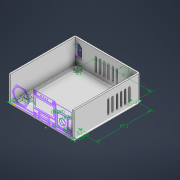
# Autodesk Inventor part: Part1
Saved by Autodesk Inventor 2021 (Build 250183000, 183)
## iProperties
Created: 2022-12-02
Part Number: Part1
Material: Generic
Document SubType Name: Modeling
Designer: Martin Adytia
Density: 1 g/cm^3
Appearance: Default
Author: Martin Adytia
Autodesk Inventor part; units mm, degrees
ref_plane "YZ Plane" through (0, 0, 0) normal (1, 0, 0) x (0, 1, 0)
ref_plane "XZ Plane" through (0, 0, 0) normal (0, 1, 0) x (-1, 0, 0)
ref_plane "XY Plane" through (0, 0, 0) normal (0, 0, 1) x (1, 0, 0)
sketch "Sketch1" plane through (0, 0, 0) normal (0, 1, 0) x (-1, 0, 0)
  line L0 (0, 0) -> (-70, 0)
  line L1 (-70, 0) -> (-70, -67.3)
  line L2 (-70, -67.3) -> (0, -67.3)
  line L3 (0, -67.3) -> (0, 0)
  line L4 (-70, -67.3) -> (-70, -64.3)
  circle A0 centre (-67, -64.3) radius 1.55
  line L5 (0, -67.3) -> (0, -64.3)
  line L6 (0, -64.3) -> (-2, -64.3)
  circle A1 centre (-2, -64.3) radius 1.55
  line L7 (0, 0) -> (4, 0)
  line L8 (-70, 0) -> (-70, 9)
  line L9 (-70, -67.3) -> (-71, -67.3)
  line L10 (-71, -67.3) -> (-71, 9)
  line L11 (-71, 9) -> (-70, 9)
  line L12 (-70, 9) -> (-70, -67.3)
  line L13 (-71, -67.3) -> (0, -67.3)
  line L14 (0, -67.3) -> (0, -68.3)
  line L15 (0, -68.3) -> (-71, -68.3)
  line L16 (-71, -68.3) -> (-71, -67.3)
  line L17 (4, 0) -> (5, 0)
  line L18 (5, 0) -> (5, -68.3)
  line L19 (5, -68.3) -> (4, -68.3)
  line L20 (4, -68.3) -> (4, 0)
  line L21 (0, -67.3) -> (4, -67.3)
  line L22 (4, -68.3) -> (0, -68.3)
  line L23 (-71, 9) -> (5, 9)
  line L24 (5, 9) -> (5, 8)
  line L25 (5, 8) -> (-71, 8)
  line L26 (-71, 8) -> (-71, 9)
  line L27 (5, 0) -> (4, 0)
  line L28 (4, 0) -> (4, 8)
  line L29 (4, 8) -> (5, 8)
  line L30 (5, 8) -> (5, 0)
  line L31 (5, -68.3) -> (-71, -68.3)
  line L32 (-71, -68.3) -> (-71, -70.3)
  line L33 (-71, -70.3) -> (5, -70.3)
  line L34 (5, -70.3) -> (5, -68.3)
  line L35 (-71, -70.3) -> (-73, -70.3)
  line L36 (-73, -70.3) -> (-73, 9)
  line L37 (-73, 9) -> (-71, 9)
  line L38 (-71, 9) -> (-71, -70.3)
  line L39 (-73, 9) -> (5, 9)
  line L40 (5, 9) -> (5, 11)
  line L41 (5, 11) -> (-73, 11)
  line L42 (-73, 11) -> (-73, 9)
  line L43 (5, 11) -> (7, 11)
  line L44 (7, 11) -> (7, -70.3)
  line L45 (7, -70.3) -> (5, -70.3)
  line L46 (5, -70.3) -> (5, 11)
  circle A2 centre (-2, -64.3) radius 3
  circle A3 centre (-67, -64.3) radius 3
  circle A4 centre (-66.9693, -3.0346) radius 1.55
  circle A5 centre (-66.9693, -3.0346) radius 3
  circle A6 centre (-2.0948, -2.9942) radius 1.55
  circle A7 centre (-2.0948, -2.9942) radius 3
  point P0 (-69, -63.3)
  dimension "d0" = 70
  dimension "d1" = 67.3
  dimension "d2" = 3
  dimension "d3" = 3.1
  dimension "d4" = 3
  dimension "d5" = 2
  dimension "d6" = 3.1
  dimension "d7" = 4
  dimension "d8" = 9
  dimension "d9" = 1
  dimension "d10" = 1
  dimension "d11" = 1
  dimension "d12" = 1
  dimension "d13" = 2
  dimension "d14" = 2
  dimension "d15" = 2
  dimension "d16" = 2
  dimension "d62" = 3.1
  dimension "d63" = 6
  dimension "d64" = 3.1
  dimension "d65" = 6
  constraints: 94 end point, 21 parallel, 12 perpendicular, 11 horizontal, 7 centre point, 7 point on line, 5 coincident, 1 horizontal alignment, 1 vertical, 2 other
  measures "d0" distance of L2.end L1.end
  measures "d1" distance of L1.end L0.end
  measures "d2" distance of L1.end L4.end
  measures "d3" diameter of A0
  measures "d4" distance of L2.end L5.end
  measures "d5" distance of L5.end L6.end
  measures "d6" diameter of A1
  measures "d7" distance of L0.start L7.end
  measures "d8" distance of L0.end L8.end
  measures "d9" distance of L10.end L11.end
  measures "d10" distance of L13.end L14.end
  measures "d11" distance of L18.end L19.end
  measures "d12" distance of L23.end L24.end
  measures "d13" distance of L32.end L31.end
  measures "d14" distance of L36.end L37.end
  measures "d15" distance of L40.end L39.end
  measures "d16" distance of L44.end L45.end
  measures "d62" diameter of A4
  measures "d63" diameter of A5
  measures "d64" diameter of A6
  measures "d65" diameter of A7
extrude "Extrusion2" add sketch "Sketch1" against normal blind 2 contours L3 A7 L0 | L7 L20 L21 L3 A2 A7 | L0 A7 L8 L25 L28 L7 | A7 L3 L0 | L0 A7 | A7 L3 | L28 L25 L30 L17 | L17 L18 L19 L20 | A7 L3 A2 L2 A3 L1 L0 | L30 L24 L40 L43 L44 L45 L34 L18 | L20 L22 L14 L21 | L25 L8 L23 L24 | L1 L9 L10 L25 L8 | A2 L3 | L3 A2 | L34 L33 L32 L15 L22 L19 | L14 L15 L16 L9 L2 | L2 A2 L3 | L25 L10 L11 L8 | A3 L2 L1 | A3 | L23 L11 L37 L42 L41 L40 | L10 L16 L32 L35 L36 L37 | A0 | A1 | A4 | A5 | A6
extrude "Extrusion3" add sketch "Sketch1" along normal blind 3 contours A2 L3 | L3 A2 | A3
extrude "Extrusion4" cut sketch "Sketch1" against normal blind 1 contours A0 | A1
fillet "Fillet1" radius 1 1 edges at (70, 0, -64.3)
fillet "Fillet2" radius 1 1 edges at (5, 0, -64.3)
extrude "Extrusion5" add sketch "Sketch1" along normal blind 30 contours L30 L24 L40 L43 L44 L45 L34 L18 | L34 L33 L32 L15 L22 L19 | L23 L11 L37 L42 L41 L40 | L10 L16 L32 L35 L36 L37
sketch "Sketch2" plane through (-7, -2, 11) normal (0, 0, 1) x (1, 0, 0)
  line L0 (71.2558, 20.3181) -> (59.4702, 20.3181)
  line L1 (59.4702, 20.3181) -> (59.4702, 18.5401)
  line L2 (59.4702, 15.3651) -> (59.4702, 10.5391)
  line L3 (59.4702, 7.3641) -> (59.4702, 6.6021)
  line L4 (59.4702, 6.6021) -> (71.2558, 6.6021)
  line L5 (71.2558, 6.6021) -> (71.2558, 7.3641)
  line L6 (71.2558, 10.5391) -> (71.2558, 15.3651)
  line L7 (71.2558, 18.5401) -> (71.2558, 20.3181)
  line L8 (77.0216, 28.7521) -> (57.6922, 28.7521)
  line L9 (57.6922, 28.7521) -> (57.6922, 2.3361)
  line L10 (57.6922, 2.3361) -> (77.0216, 2.3361)
  line L11 (77.0216, 2.3361) -> (77.0216, 28.7521)
  circle A0 centre (74.5578, 22.0211) radius 1.5
  circle A1 centre (74.5578, 8.1019) radius 1.5
  circle A2 centre (65.363, 12.9521) radius 3.4544
  line L12 (54.1324, 12.5617) -> (54.1324, 23.7817)
  line L13 (54.1324, 23.7817) -> (32.5724, 23.7817)
  line L14 (32.5724, 23.7817) -> (32.5724, 12.5617)
  line L15 (32.5724, 12.5617) -> (54.1324, 12.5617)
  line L16 (56.1024, 10.9717) -> (56.1024, 25.3717)
  line L17 (56.1024, 25.3717) -> (30.6024, 25.3717)
  line L18 (30.6024, 25.3717) -> (30.6024, 10.9717)
  line L19 (30.6024, 10.9717) -> (56.1024, 10.9717)
  line L20 (54.1324, 23.7817) -> (54.1324, 12.5617)
  line L21 (54.1324, 12.5617) -> (32.5724, 12.5617)
  line L22 (32.5724, 12.5617) -> (32.5724, 23.7817)
  line L23 (32.5724, 23.7817) -> (54.1324, 23.7817)
  line L24 (35.8555, 8.9917) -> (49.8555, 8.9917)
  line L25 (49.8555, 8.9917) -> (49.8555, 7.9917)
  line L26 (49.8555, 7.9917) -> (47.8555, 7.9917)
  line L27 (47.8555, 7.9917) -> (47.8554, 6.6117)
  line L28 (47.8554, 6.6117) -> (56.6024, 6.6117)
  line L29 (56.6024, 25.8717) -> (56.6024, 6.6117)
  line L30 (30.1024, 25.8717) -> (56.6024, 25.8717)
  line L31 (30.1024, 6.6117) -> (30.1024, 25.8717)
  line L32 (30.1024, 6.6117) -> (37.8601, 6.6117)
  line L33 (37.8601, 6.6117) -> (37.8601, 7.9917)
  line L34 (37.8601, 7.9917) -> (35.8555, 7.9917)
  line L35 (35.8555, 7.9917) -> (35.8555, 8.9917)
  line L36 (30.6024, 25.3717) -> (56.1024, 25.3717)
  line L37 (56.1024, 25.3717) -> (56.1024, 10.9717)
  line L38 (56.1024, 10.9717) -> (30.6024, 10.9717)
  line L39 (30.6024, 10.9717) -> (30.6024, 25.3717)
  arc A3 (31.8024, 2.3117) -> (30.0024, 4.1117) centre (31.8024, 4.1117) ccw
  line L40 (31.8024, 2.3117) -> (35.8555, 2.3117)
  line L41 (35.8555, 2.3117) -> (35.8555, 4.3117)
  line L42 (49.8555, 4.3117) -> (35.8555, 4.3117)
  line L43 (49.8555, 4.3117) -> (49.8555, 2.3117)
  line L44 (49.8555, 2.3117) -> (54.9024, 2.3117)
  arc A4 (56.7024, 4.1117) -> (54.9024, 2.3117) centre (54.9024, 4.1117) ccw
  line L45 (56.7024, 30.1717) -> (56.7024, 4.1117)
  line L46 (30.0024, 30.1717) -> (56.7024, 30.1717)
  line L47 (30.0024, 30.1717) -> (30.0024, 4.1117)
  circle A5 centre (42.0824, 27.8217) radius 0.5
  circle A6 centre (44.6224, 27.8217) radius 0.5
  circle A7 centre (47.1624, 27.8217) radius 0.5
  circle A8 centre (39.5424, 27.8217) radius 0.5
  circle A9 centre (54.9024, 27.6717) radius 1
  circle A10 centre (31.8024, 27.6717) radius 1
  line L48 (56.6024, 10.3717) -> (56.6024, 25.8717)
  line L49 (30.1024, 10.3717) -> (56.6024, 10.3717)
  line L50 (30.1024, 25.8717) -> (30.1024, 10.3717)
  line L51 (56.6024, 25.8717) -> (30.1024, 25.8717)
  circle A11 centre (31.8024, 4.1117) radius 1.8
  line L52 (30.0024, 2.3117) -> (31.8024, 2.3117)
  line L53 (30.0024, 4.1117) -> (30.0024, 2.3117)
  line L54 (54.9024, 2.3117) -> (56.7024, 2.3117)
  line L55 (56.7024, 4.1117) -> (56.7024, 2.3117)
  circle A12 centre (54.9024, 4.1117) radius 1.8
  circle A13 centre (54.9024, 27.6717) radius 1.8
  circle A14 centre (31.8024, 27.6717) radius 1.8
  line L56 (37.8601, 6.6117) -> (37.8601, 2.3117)
  line L57 (47.8554, 6.6117) -> (37.8601, 6.6117)
  line L58 (37.8601, 6.6117) -> (37.8601, 2.3117)
  line L59 (47.8554, 2.3117) -> (37.8601, 2.3117)
  line L60 (47.8554, 2.3117) -> (47.8554, 6.6117)
  line L61 (36.8554, 6.6117) -> (36.8554, 2.3318)
  line L62 (36.8554, 2.3318) -> (48.8554, 2.3318)
  line L63 (48.8554, 2.3318) -> (48.8554, 6.6117)
  line L64 (48.8554, 6.6117) -> (36.8554, 6.6117)
  line L65 (48.8554, 2.3318) -> (48.8554, 6.6117)
  circle A15 centre (14.6189, 15.1235) radius 9.5
  circle A16 centre (14.6189, 15.1235) radius 8.4463
  line L66 (7.7436, 8.0317) -> (5.0396, 12.7153)
  line L67 (17.3229, 5.6235) -> (11.9148, 5.6235)
  line L68 (9.1386, 5.6235) -> (11.9148, 5.6235)
  line L69 (7.7436, 8.0317) -> (9.1317, 5.6275)
  line L70 (20.106, 5.6275) -> (21.4941, 8.0317)
  line L71 (17.3229, 5.6235) -> (20.0991, 5.6235)
  line L72 (24.1981, 12.7153) -> (21.4941, 8.0317)
  line L73 (24.1981, 12.7153) -> (25.5862, 15.1195)
  line L74 (25.5862, 15.1275) -> (24.1981, 17.5317)
  line L75 (21.4941, 22.2153) -> (24.1981, 17.5317)
  line L76 (21.4941, 22.2153) -> (20.106, 24.6195)
  line L77 (20.0991, 24.6235) -> (17.3229, 24.6235)
  line L78 (11.9148, 24.6235) -> (17.3229, 24.6235)
  line L79 (11.9148, 24.6235) -> (9.1386, 24.6235)
  line L80 (9.1317, 24.6195) -> (7.7436, 22.2153)
  line L81 (5.0396, 17.5317) -> (7.7436, 22.2153)
  line L82 (5.0396, 17.5317) -> (3.6515, 15.1275)
  line L83 (3.6515, 15.1195) -> (5.0396, 12.7153)
  line L84 (59.4702, 20.3181) -> (59.4702, 20.8181)
  line L85 (59.4702, 20.3181) -> (59.9702, 20.3181) construction
  line L86 (71.2558, 20.3181) -> (71.7558, 20.3181)
  line L87 (71.2558, 20.3181) -> (71.7558, 20.3181) construction
  line L88 (71.2558, 6.6021) -> (71.2558, 6.1021)
  line L89 (59.4702, 6.6021) -> (58.9702, 6.6021)
  line L90 (59.4702, 20.8181) -> (71.7558, 20.8181)
  line L91 (71.7558, 20.8181) -> (71.7558, 6.1021)
  line L92 (71.7558, 6.1021) -> (58.9702, 6.1021)
  line L93 (58.9702, 6.1021) -> (58.9702, 20.8181)
  line L94 (58.9702, 20.8181) -> (59.4702, 20.8181)
  circle A17 centre (65.363, 12.9521) radius 3.8
  line L95 (71.2558, 18.5401) -> (71.2558, 15.3651)
  line L96 (71.2558, 10.5391) -> (71.2558, 7.3641)
  line L97 (59.4702, 10.5391) -> (59.4702, 7.3641)
  line L98 (59.4702, 18.5401) -> (59.4702, 15.3651)
  line L99 (57.6922, 22.6169) -> (73.0578, 22.6169)
  line L100 (73.0578, 22.6169) -> (73.0578, 4.7047)
  line L101 (73.0578, 4.7047) -> (57.6922, 4.7047)
  line L102 (57.6922, 4.7047) -> (57.6922, 22.6169)
  circle A18 centre (31.8024, 4.1117) radius 1
  circle A19 centre (54.9024, 4.1117) radius 1
  point P0 (7, 2)
  point P1 (45.1104, -3.166)
  point P2 (36.8554, 4.3117)
  point P3 (48.8554, 4.3117)
  point P4 (37.8601, 2.3318)
  point P5 (47.8554, 2.3318)
  dimension "d31" = 0.5
  dimension "d32" = 90
  dimension "d33" = 0.5
  dimension "d34" = 0
  dimension "d35" = 0.5
  dimension "d36" = 0.5
  dimension "d37" = 7.6
  constraints: 206 end point, 20 centre point, 6 horizontal, 5 perpendicular, 4 coincident, 4 point on circle, 3 collinear, 3 parallel, 2 equal length, 2 point on line, 2 vertical
  measures "d31" distance of L0.end L84.end
  measures "d32" angle of L85 L84
  measures "d33" distance of L0.start L86.end
  measures "d34" distance between parallel lines of L86 L87
  measures "d35" distance of L4.end L88.end
  measures "d36" distance of L3.end L89.end
  measures "d37" diameter of A17
extrude "Extrusion6" cut sketch "Sketch2" against normal blind 10 contours A16
extrude "Extrusion7" cut sketch "Sketch2" against normal blind 10 contours A2 | A17
extrude "Extrusion8" add sketch "Sketch2" against normal blind 8 contours L86 L91 L92 L88 L5 L96 L6 L95 L7 | L0 L84 L90 L91 L86 | L1 L98 L2 L97 L3 L89 L93 L94 L84 | L92 L93 L89 L4 L88 | L99 L100 L101 L9
extrude "Extrusion9" cut sketch "Sketch2" against normal blind 8 contours L15 L14 L13 L12 | L19 L18 L17 L16
extrude "Extrusion13" add sketch "Sketch2" against normal blind 5 contours L15 L14 L13 L12 | L19 L18 L17 L16 | L35 L34 L33 L32 L31 L49 L29 L28 L27 L26 L25 L24 | L24 L25 L26 L27 L57 L33 L34 L35 | L56 L42 L61 L32 | L57 L60 L42 L56 | L28 L63 L42 L60 | L61 L42 L41 L40 A3 L47 A14 L30 L31 L32 | L56 L62 L61 L42 | L42 L60 L62 L56 | L28 L29 L30 A13 L45 A4 L44 L43 L42 L63 | L42 L63 L62 L60 | L62 L60 L59 L56 | L31 L30 L29 L49 | A14 L47 L46 L45 A13 L30 | A14 | A11 A3 | L52 L53 A11 | A13 | A12 L55 L54 | A4 A12 | A5 | A6 | A7 | A8 | A9 | A10 | A18 | A19
extrude "Extrusion14" cut sketch "Sketch2" against normal blind 5 contours L15 L14 L13 L12 | L19 L18 L17 L16
extrude "Extrusion15" cut sketch "Sketch2" against normal blind 5 contours A9
extrude "Extrusion16" cut sketch "Sketch2" against normal blind 5 contours A10 | A18 | A19
extrude "Extrusion17" add sketch "Sketch2" against normal blind 2 contours A9 | A10 | A18 | A19
sketch "Sketch3" plane through (0, 30, 0) normal (0, 1, 0) x (1, 0, 0)
  line L0 (71, -9) -> (71, 64.3) projected
  line L1 (-5, -11) -> (71, -11)
  line L2 (71, -11) -> (71, 0)
  line L3 (71, 0) -> (-5, 0)
  line L4 (-5, 0) -> (-5, -11)
  point P0 (0, 0)
  constraints: 8 end point, 2 parallel, 1 horizontal, 1 perpendicular, 1 point on line
extrude "Extrusion18" cut sketch "Sketch3" against normal blind 30
extrude "Extrusion19" add sketch "Sketch1" along normal blind 3 contours A7 L3 L0 | L0 A7 | A7 L3 | A4 | A5 | A6 picked at (-0.1816, -2.9942)
extrude "Extrusion20" cut sketch "Sketch1" along normal blind 3 contours A6
extrude "Extrusion21" cut sketch "Sketch1" against normal blind 1 contours A6
extrude "Extrusion22" cut sketch "Sketch1" along normal blind 3 contours A4
extrude "Extrusion23" cut sketch "Sketch1" against normal blind 1 contours A4
fillet "Fillet3" radius 2 2 edges at (5.0948, 0, -2.9942) (69.9693, 0, -3.0346)
sketch "Sketch4" plane through (73, -2, -70.3) normal (0, 0, -1) x (-1, 0, 0)
  line L0 (77.9837, 11.3959) -> (77.9837, 23.7773)
  arc A0 (77.9837, 23.7773) -> (77.9105, 23.9541) centre (77.7337, 23.7773) ccw
  line L1 (77.9105, 23.9541) -> (75.0569, 26.8076)
  arc A1 (75.0569, 26.8076) -> (74.8801, 26.8809) centre (74.8801, 26.6309) ccw
  line L2 (74.8801, 26.8809) -> (72.9592, 26.8809)
  line L3 (72.7825, 26.8076) -> (69.8557, 23.8809)
  arc A2 (72.9592, 26.8809) -> (72.7825, 26.8076) centre (72.9592, 26.6309) ccw
  line L4 (70.1057, 11.1459) -> (77.7337, 11.1459)
  arc A3 (77.7337, 11.1459) -> (77.9837, 11.3959) centre (77.7337, 11.3959) ccw
  arc A4 (69.8557, 11.3959) -> (70.1057, 11.1459) centre (70.1057, 11.3959) ccw
  line L5 (69.8557, 23.8809) -> (69.8557, 11.3959)
  line L6 (80, 0) -> (80, 32) projected
  line L7 (80, 21.6857) -> (78, 21.6857)
  line L8 (78, 2) -> (78, 32) projected
  line L9 (37, 24) -> (37, 24)
  line L10 (38, 23) -> (38, 8)
  line L11 (37, 7) -> (37, 7)
  line L12 (36, 8) -> (36, 23)
  line L13 (42, 24) -> (42, 24)
  line L14 (43, 23) -> (43, 8)
  line L15 (42, 7) -> (42, 7)
  line L16 (41, 8) -> (41, 23)
  line L17 (47.2198, 23.9651) -> (47.2198, 23.9651)
  line L18 (48.2198, 22.9651) -> (48.2198, 7.9651)
  line L19 (47.2198, 6.9651) -> (47.2198, 6.9651)
  line L20 (46.2198, 7.9651) -> (46.2198, 22.9651)
  line L21 (52.2198, 23.9651) -> (52.2198, 23.9651)
  line L22 (53.2198, 22.9651) -> (53.2198, 7.9651)
  line L23 (52.2198, 6.9651) -> (52.2198, 6.9651)
  line L24 (51.2198, 7.9651) -> (51.2198, 22.9651)
  line L25 (32.3855, 23.0054) -> (32.3855, 8.0054)
  line L26 (31.3855, 24.0054) -> (31.3855, 24.0054)
  line L27 (31.3855, 7.0054) -> (31.3855, 7.0054)
  line L28 (30.3855, 8.0054) -> (30.3855, 23.0054)
  line L29 (27.3855, 23.0054) -> (27.3855, 8.0054)
  line L30 (26.3855, 24.0054) -> (26.3855, 24.0054)
  line L31 (26.3855, 7.0054) -> (26.3855, 7.0054)
  line L32 (25.3855, 8.0054) -> (25.3855, 23.0054)
  arc A5 (26.3855, 24.0054) -> (25.3855, 23.0054) centre (26.3855, 23.0054) ccw
  arc A6 (27.3855, 23.0054) -> (26.3855, 24.0054) centre (26.3855, 23.0054) ccw
  arc A7 (25.3855, 8.0054) -> (26.3855, 7.0054) centre (26.3855, 8.0054) ccw
  arc A8 (26.3855, 7.0054) -> (27.3855, 8.0054) centre (26.3855, 8.0054) ccw
  arc A9 (30.3855, 8.0054) -> (31.3855, 7.0054) centre (31.3855, 8.0054) ccw
  arc A10 (31.3855, 7.0054) -> (32.3855, 8.0054) centre (31.3855, 8.0054) ccw
  arc A11 (32.3855, 23.0054) -> (31.3855, 24.0054) centre (31.3855, 23.0054) ccw
  arc A12 (31.3855, 24.0054) -> (30.3855, 23.0054) centre (31.3855, 23.0054) ccw
  arc A13 (37, 24) -> (36, 23) centre (37, 23) ccw
  arc A14 (38, 23) -> (37, 24) centre (37, 23) ccw
  arc A15 (36, 8) -> (37, 7) centre (37, 8) ccw
  arc A16 (37, 7) -> (38, 8) centre (37, 8) ccw
  arc A17 (41, 8) -> (42, 7) centre (42, 8) ccw
  arc A18 (42, 7) -> (43, 8) centre (42, 8) ccw
  arc A19 (43, 23) -> (42, 24) centre (42, 23) ccw
  arc A20 (42, 24) -> (41, 23) centre (42, 23) ccw
  arc A21 (47.2198, 23.9651) -> (46.2198, 22.9651) centre (47.2198, 22.9651) ccw
  arc A22 (48.2198, 22.9651) -> (47.2198, 23.9651) centre (47.2198, 22.9651) ccw
  arc A23 (46.2198, 7.9651) -> (47.2198, 6.9651) centre (47.2198, 7.9651) ccw
  arc A24 (47.2198, 6.9651) -> (48.2198, 7.9651) centre (47.2198, 7.9651) ccw
  arc A25 (51.2198, 7.9651) -> (52.2198, 6.9651) centre (52.2198, 7.9651) ccw
  arc A26 (52.2198, 6.9651) -> (53.2198, 7.9651) centre (52.2198, 7.9651) ccw
  arc A27 (53.2198, 22.9651) -> (52.2198, 23.9651) centre (52.2198, 22.9651) ccw
  arc A28 (52.2198, 23.9651) -> (51.2198, 22.9651) centre (52.2198, 22.9651) ccw
  point P0 (73, 2)
  point P1 (73.9221, 19.0174)
  point P2 (41, 24)
  point P3 (43, 7)
  point P4 (51.2198, 23.9651)
  point P5 (53.2198, 6.9651)
  point P6 (32.3855, 7.0054)
  point P7 (30.3855, 24.0054)
  point P8 (52.2198, 6.9651)
  point P9 (42, 7)
  point P10 (37, 7)
  point P11 (31.3855, 24.0054)
  point P12 (31.3855, 7.0054)
  point P13 (26.3855, 7.0054)
  dimension "d77" = 2
  dimension "d80" = 1
  constraints: 62 end point, 58 point on circle, 48 tangent, 29 centre point, 23 equal radius, 20 point on line, 12 parallel, 6 horizontal, 6 perpendicular
  measures "d77" distance of L7.start L7.end
  measures "d80" radius of A5
extrude "Extrusion24" cut sketch "Sketch4" against normal blind 2 contours A3 L4 A4 L5 L3 A2 L2 A1 L1 A0 L0
extrude "Extrusion25" cut sketch "Sketch4" against normal blind 2 contours L10 A16 A15 L12 A13 A14 | L14 A18 A17 L16 A20 A19 | L18 A24 A23 L20 A21 A22 | L22 A26 A25 L24 A28 A27 | L25 A10 A9 L28 A12 A11 | L29 A8 A7 L32 A5 A6
sketch "Sketch5" plane through (73, -2, 11) normal (1, 0, 0) x (0, 0, -1)
  line L0 (53.5678, 23) -> (53.5678, 8)
  line L1 (51.5678, 8) -> (51.5678, 23)
  line L2 (58.7235, 23) -> (58.7235, 8)
  line L3 (56.7235, 8) -> (56.7235, 23)
  line L4 (68.7007, 22.9651) -> (68.7007, 7.9651)
  line L5 (66.7007, 7.9651) -> (66.7007, 22.9651)
  line L6 (63.7007, 22.9651) -> (63.7007, 7.9651)
  line L7 (61.7007, 7.9651) -> (61.7007, 22.9651)
  line L8 (47.9904, 23.0054) -> (47.9904, 8.0054)
  line L9 (45.9904, 8.0054) -> (45.9904, 23.0054)
  line L10 (42.8842, 23.0054) -> (42.8842, 8.0054)
  line L11 (40.8842, 8.0054) -> (40.8842, 23.0054)
  arc A0 (41.8842, 24.0054) -> (40.8842, 23.0054) centre (41.8842, 23.0054) ccw
  arc A1 (42.8842, 23.0054) -> (41.8842, 24.0054) centre (41.8842, 23.0054) ccw
  arc A2 (40.8842, 8.0054) -> (41.8842, 7.0054) centre (41.8842, 8.0054) ccw
  arc A3 (41.8842, 7.0054) -> (42.8842, 8.0054) centre (41.8842, 8.0054) ccw
  arc A4 (45.9904, 8.0054) -> (46.9904, 7.0054) centre (46.9904, 8.0054) ccw
  arc A5 (46.9904, 7.0054) -> (47.9904, 8.0054) centre (46.9904, 8.0054) ccw
  arc A6 (47.9904, 23.0054) -> (46.9904, 24.0054) centre (46.9904, 23.0054) ccw
  arc A7 (46.9904, 24.0054) -> (45.9904, 23.0054) centre (46.9904, 23.0054) ccw
  arc A8 (52.5678, 24) -> (51.5678, 23) centre (52.5678, 23) ccw
  arc A9 (53.5678, 23) -> (52.5678, 24) centre (52.5678, 23) ccw
  arc A10 (51.5678, 8) -> (52.5678, 7) centre (52.5678, 8) ccw
  arc A11 (52.5678, 7) -> (53.5678, 8) centre (52.5678, 8) ccw
  arc A12 (56.7235, 8) -> (57.7235, 7) centre (57.7235, 8) ccw
  arc A13 (57.7235, 7) -> (58.7235, 8) centre (57.7235, 8) ccw
  arc A14 (58.7235, 23) -> (57.7235, 24) centre (57.7235, 23) ccw
  arc A15 (57.7235, 24) -> (56.7235, 23) centre (57.7235, 23) ccw
  arc A16 (62.7007, 23.9651) -> (61.7007, 22.9651) centre (62.7007, 22.9651) ccw
  arc A17 (63.7007, 22.9651) -> (62.7007, 23.9651) centre (62.7007, 22.9651) ccw
  arc A18 (61.7007, 7.9651) -> (62.7007, 6.9651) centre (62.7007, 7.9651) ccw
  arc A19 (62.7007, 6.9651) -> (63.7007, 7.9651) centre (62.7007, 7.9651) ccw
  arc A20 (66.7007, 7.9651) -> (67.7007, 6.9651) centre (67.7007, 7.9651) ccw
  arc A21 (67.7007, 6.9651) -> (68.7007, 7.9651) centre (67.7007, 7.9651) ccw
  arc A22 (68.7007, 22.9651) -> (67.7007, 23.9651) centre (67.7007, 22.9651) ccw
  arc A23 (67.7007, 23.9651) -> (66.7007, 22.9651) centre (67.7007, 22.9651) ccw
  point P0 (11, 2)
  point P1 (56.7235, 24)
  point P2 (58.7235, 7)
  point P3 (68.7007, 6.9651)
  point P4 (66.7007, 23.9651)
  point P5 (47.9904, 7.0054)
  point P6 (45.9904, 24.0054)
  point P7 (67.7007, 23.9651)
  point P8 (67.7007, 6.9651)
  point P9 (62.7007, 23.9651)
  point P10 (62.7007, 6.9651)
  point P11 (57.7235, 24)
  point P12 (57.7235, 7)
  point P13 (52.5678, 7)
  point P14 (52.5678, 24)
  point P15 (46.9904, 24.0054)
  point P16 (41.8842, 24.0054)
  point P17 (41.8842, 7.0054)
  dimension "d83" = 1
  constraints: 48 point on circle, 24 centre point, 24 end point, 24 tangent, 23 equal radius, 6 parallel, 6 point on line, 6 vertical, 72 other
  measures "d83" radius of A0
extrude "Extrusion26" cut sketch "Sketch5" against normal blind 2
fillet "Fillet4" radius 2 2 edges at (-7, 14, -70.3) (73, 14, -70.3)
body "Solid2"
